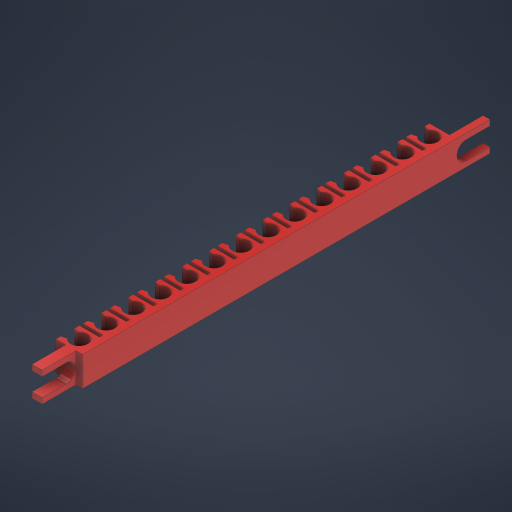
# Autodesk Inventor part: Hose Clamp
Saved by Autodesk Inventor 2024 (Build 280153000, 153)
## iProperties
Created: 2023-05-24
Part Number: Hose Clamp
Material: Generic
Document SubType Name: Modeling
Designer: cfangmeier3
Density: 1 g/cm^3
Appearance: Default
Author: cfangmeier3
Autodesk Inventor part; units mm, degrees
ref_plane "YZ Plane" through (0, 0, 0) normal (1, 0, 0) x (0, 1, 0)
ref_plane "XZ Plane" through (0, 0, 0) normal (0, 1, 0) x (-1, 0, 0)
ref_plane "XY Plane" through (0, 0, 0) normal (0, 0, 1) x (1, 0, 0)
sketch "Sketch1" plane through (0, 0, 0) normal (0, 1, 0) x (-1, 0, 0)
  line L0 (0, 71.12) -> (0, -71.12)
  line L1 (2.54, 71.12) -> (10.0965, 71.12)
  line L2 (10.0965, 71.12) -> (10.0965, 69.215)
  line L3 (10.0965, 64.135) -> (10.0965, 62.23)
  line L4 (10.0965, 69.215) -> (8.1249, 68.7234)
  line L5 (10.0965, 64.135) -> (8.1249, 64.6266)
  arc A0 (8.1249, 68.7234) -> (8.1249, 64.6266) centre (5.699, 66.675) ccw
  line L6 (10.0965, 62.23) -> (2.54, 62.23)
  line L7 (2.54, 62.23) -> (2.54, 60.96)
  line L8 (2.54, 52.07) -> (2.54, 50.8)
  line L9 (10.0965, 52.07) -> (2.54, 52.07)
  line L10 (10.0965, 53.975) -> (10.0965, 52.07)
  line L11 (10.0965, 59.055) -> (8.1249, 58.5634)
  arc A1 (8.1249, 58.5634) -> (8.1249, 54.4666) centre (5.699, 56.515) ccw
  line L12 (2.54, 60.96) -> (10.0965, 60.96)
  line L13 (10.0965, 60.96) -> (10.0965, 59.055)
  line L14 (10.0965, 53.975) -> (8.1249, 54.4666)
  line L15 (2.54, 41.91) -> (2.54, 40.64)
  line L16 (10.0965, 41.91) -> (2.54, 41.91)
  line L17 (10.0965, 43.815) -> (10.0965, 41.91)
  line L18 (10.0965, 48.895) -> (8.1249, 48.4034)
  arc A2 (8.1249, 48.4034) -> (8.1249, 44.3066) centre (5.699, 46.355) ccw
  line L19 (2.54, 50.8) -> (10.0965, 50.8)
  line L20 (10.0965, 50.8) -> (10.0965, 48.895)
  line L21 (10.0965, 43.815) -> (8.1249, 44.3066)
  line L22 (2.54, 31.75) -> (2.54, 30.48)
  line L23 (10.0965, 31.75) -> (2.54, 31.75)
  line L24 (10.0965, 33.655) -> (10.0965, 31.75)
  line L25 (10.0965, 38.735) -> (8.1249, 38.2434)
  arc A3 (8.1249, 38.2434) -> (8.1249, 34.1466) centre (5.699, 36.195) ccw
  line L26 (2.54, 40.64) -> (10.0965, 40.64)
  line L27 (10.0965, 40.64) -> (10.0965, 38.735)
  line L28 (10.0965, 33.655) -> (8.1249, 34.1466)
  line L29 (2.54, 21.59) -> (2.54, 20.32)
  line L30 (10.0965, 21.59) -> (2.54, 21.59)
  line L31 (10.0965, 23.495) -> (10.0965, 21.59)
  line L32 (10.0965, 28.575) -> (8.1249, 28.0834)
  arc A4 (8.1249, 28.0834) -> (8.1249, 23.9866) centre (5.699, 26.035) ccw
  line L33 (2.54, 30.48) -> (10.0965, 30.48)
  line L34 (10.0965, 30.48) -> (10.0965, 28.575)
  line L35 (10.0965, 23.495) -> (8.1249, 23.9866)
  line L36 (2.54, 11.43) -> (2.54, 10.16)
  line L37 (10.0965, 11.43) -> (2.54, 11.43)
  line L38 (10.0965, 13.335) -> (10.0965, 11.43)
  line L39 (10.0965, 18.415) -> (8.1249, 17.9234)
  arc A5 (8.1249, 17.9234) -> (8.1249, 13.8266) centre (5.699, 15.875) ccw
  line L40 (2.54, 20.32) -> (10.0965, 20.32)
  line L41 (10.0965, 20.32) -> (10.0965, 18.415)
  line L42 (10.0965, 13.335) -> (8.1249, 13.8266)
  line L43 (2.54, 1.27) -> (2.54, 0)
  line L44 (10.0965, 1.27) -> (2.54, 1.27)
  line L45 (10.0965, 3.175) -> (10.0965, 1.27)
  line L46 (10.0965, 8.255) -> (8.1249, 7.7634)
  arc A6 (8.1249, 7.7634) -> (8.1249, 3.6666) centre (5.699, 5.715) ccw
  line L47 (2.54, 10.16) -> (10.0965, 10.16)
  line L48 (10.0965, 10.16) -> (10.0965, 8.255)
  line L49 (10.0965, 3.175) -> (8.1249, 3.6666)
  line L50 (2.54, -8.89) -> (2.54, -10.16)
  line L51 (10.0965, -8.89) -> (2.54, -8.89)
  line L52 (10.0965, -6.985) -> (10.0965, -8.89)
  line L53 (10.0965, -1.905) -> (8.1249, -2.3966)
  arc A7 (8.1249, -2.3966) -> (8.1249, -6.4934) centre (5.699, -4.445) ccw
  line L54 (2.54, 0) -> (10.0965, 0)
  line L55 (10.0965, 0) -> (10.0965, -1.905)
  line L56 (10.0965, -6.985) -> (8.1249, -6.4934)
  line L57 (2.54, -19.05) -> (2.54, -20.32)
  line L58 (10.0965, -19.05) -> (2.54, -19.05)
  line L59 (10.0965, -17.145) -> (10.0965, -19.05)
  line L60 (10.0965, -12.065) -> (8.1249, -12.5566)
  arc A8 (8.1249, -12.5566) -> (8.1249, -16.6534) centre (5.699, -14.605) ccw
  line L61 (2.54, -10.16) -> (10.0965, -10.16)
  line L62 (10.0965, -10.16) -> (10.0965, -12.065)
  line L63 (10.0965, -17.145) -> (8.1249, -16.6534)
  line L64 (2.54, -29.21) -> (2.54, -30.48)
  line L65 (10.0965, -29.21) -> (2.54, -29.21)
  line L66 (10.0965, -27.305) -> (10.0965, -29.21)
  line L67 (10.0965, -22.225) -> (8.1249, -22.7166)
  arc A9 (8.1249, -22.7166) -> (8.1249, -26.8134) centre (5.699, -24.765) ccw
  line L68 (2.54, -20.32) -> (10.0965, -20.32)
  line L69 (10.0965, -20.32) -> (10.0965, -22.225)
  line L70 (10.0965, -27.305) -> (8.1249, -26.8134)
  line L71 (2.54, -39.37) -> (2.54, -40.64)
  line L72 (10.0965, -39.37) -> (2.54, -39.37)
  line L73 (10.0965, -37.465) -> (10.0965, -39.37)
  line L74 (10.0965, -32.385) -> (8.1249, -32.8766)
  arc A10 (8.1249, -32.8766) -> (8.1249, -36.9734) centre (5.699, -34.925) ccw
  line L75 (2.54, -30.48) -> (10.0965, -30.48)
  line L76 (10.0965, -30.48) -> (10.0965, -32.385)
  line L77 (10.0965, -37.465) -> (8.1249, -36.9734)
  line L78 (2.54, -49.53) -> (2.54, -50.8)
  line L79 (10.0965, -49.53) -> (2.54, -49.53)
  line L80 (10.0965, -47.625) -> (10.0965, -49.53)
  line L81 (10.0965, -42.545) -> (8.1249, -43.0366)
  arc A11 (8.1249, -43.0366) -> (8.1249, -47.1334) centre (5.699, -45.085) ccw
  line L82 (2.54, -40.64) -> (10.0965, -40.64)
  line L83 (10.0965, -40.64) -> (10.0965, -42.545)
  line L84 (10.0965, -47.625) -> (8.1249, -47.1334)
  line L85 (2.54, -59.69) -> (2.54, -60.96)
  line L86 (10.0965, -59.69) -> (2.54, -59.69)
  line L87 (10.0965, -57.785) -> (10.0965, -59.69)
  line L88 (10.0965, -52.705) -> (8.1249, -53.1966)
  arc A12 (8.1249, -53.1966) -> (8.1249, -57.2934) centre (5.699, -55.245) ccw
  line L89 (2.54, -50.8) -> (10.0965, -50.8)
  line L90 (10.0965, -50.8) -> (10.0965, -52.705)
  line L91 (10.0965, -57.785) -> (8.1249, -57.2934)
  line L92 (2.54, -69.85) -> (2.54, -71.12)
  line L93 (10.0965, -69.85) -> (2.54, -69.85)
  line L94 (10.0965, -67.945) -> (10.0965, -69.85)
  line L95 (10.0965, -62.865) -> (8.1249, -63.3566)
  arc A13 (8.1249, -63.3566) -> (8.1249, -67.4534) centre (5.699, -65.405) ccw
  line L96 (2.54, -60.96) -> (10.0965, -60.96)
  line L97 (10.0965, -60.96) -> (10.0965, -62.865)
  line L98 (10.0965, -67.945) -> (8.1249, -67.4534)
  line L99 (0, 71.12) -> (2.54, 71.12)
  line L100 (6.35, 71.12) -> (2.54, 71.12)
  line L101 (2.54, 71.12) -> (2.54, 83.82)
  line L102 (2.54, 83.82) -> (6.35, 83.82)
  line L103 (6.35, 83.82) -> (6.35, 71.12)
  line L104 (2.54, -71.12) -> (2.54, -82.55)
  line L105 (2.54, -82.55) -> (0, -82.55)
  line L106 (0, -82.55) -> (0, -71.12)
  point P0 (0, 0)
  dimension "d1" = 7.5565
  dimension "d5" = 104
  dimension "d6" = 104
  dimension "d7" = 3.175
  dimension "d8" = 2.032
  dimension "d9" = 2.54
  dimension "d10" = 1.27
  dimension "d11" = 8.89
  dimension "d12" = 1.905
  dimension "d16" = 10.16
  dimension "d25" = 142.24
  dimension "d26" = 71.12
  dimension "d27" = 12.7
  dimension "d28" = 3.81
  dimension "d29" = 2.54
  dimension "d41" = 12.7
  constraints: 214 end point, 28 point on circle, 14 centre point, 6 vertical, 4 horizontal, 3 perpendicular, 2 equal length, 2 horizontal alignment, 2 parallel, 1 midpoint, 1 point on line, 1 vertical alignment, 234 other
  measures "d1" distance of L1.start L1.end
  measures "d5" angle of L4 L2
  measures "d6" angle of L5 L3
  measures "d7" radius of A0
  measures "d8" distance of L2.end L4.end
  measures "d9" distance from line of L0 L6.end
  measures "d10" distance of L6.end L7.end
  measures "d11" distance between parallel lines of L1 L6
  measures "d12" distance of L1.end L2.end
  measures "d16" distance of L7.end L8.end
  measures "d25" distance of L0.start L0.end
  measures "d26" distance of L0.end point (0, 0)
  measures "d27" distance of L102.end L100.start
  measures "d28" distance of L101.end L102.end
  measures "d29" distance of L0.start L100.end
  measures "d41" distance between parallel lines of L105 L93
extrude "Extrusion1" add sketch "Sketch1" along normal blind 11.1125
sketch "Sketch3" plane through (0, 0, 71.12) normal (1, 0, 0) x (0, 0, -1)
  line L0 (162.687, 5.5563) -> (144.653, 5.5562) construction
  line L1 (162.687, 8.9853) -> (144.653, 8.9853)
  line L2 (144.653, 2.1272) -> (162.687, 2.1273)
  arc A0 (162.687, 2.1273) -> (162.687, 8.9853) centre (162.687, 5.5563) ccw
  arc A1 (144.653, 8.9853) -> (144.653, 2.1272) centre (144.653, 5.5562) ccw
  line L3 (153.67, 0) -> (153.67, 11.1125) projected
  line L4 (0, 11.1125) -> (153.67, 11.1125) projected
  line L5 (-21.717, 5.5563) -> (-3.683, 5.5563) construction
  line L6 (-21.717, 2.1273) -> (-3.683, 2.1273)
  line L7 (-3.683, 8.9853) -> (-21.717, 8.9852)
  arc A2 (-21.717, 8.9852) -> (-21.717, 2.1273) centre (-21.717, 5.5563) ccw
  arc A3 (-3.683, 2.1273) -> (-3.683, 8.9853) centre (-3.683, 5.5563) ccw
  line L8 (-12.7, 0) -> (-12.7, 11.1125) projected
  point P0 (71.12, 0)
  point P1 (153.67, 5.5563)
  point P2 (-12.7, 5.5563)
  point P3 (-12.7, 8.9853)
  point P4 (-12.7, 2.1273)
  point P5 (153.67, 2.1273)
  point P6 (153.67, 8.9853)
  dimension "d45" = 11.1125
  dimension "d46" = 5.5563
  dimension "d47" = 9.017
  dimension "d48" = 9.017
  dimension "d49" = 6.858
  dimension "d50" = 6.858
  constraints: 16 end point, 8 point on circle, 8 tangent, 4 centre point, 3 midpoint, 2 horizontal, 2 parallel, 1 collinear, 1 horizontal alignment
  measures "d45" distance of L3.start L3.end
  measures "d46" distance from line of L4 point (153.67, 5.556)
  measures "d47" distance from line of L3 L0.end
  measures "d48" distance from line of L8 L5.end
  measures "d49" distance between parallel lines of L1 L2
  measures "d50" distance between parallel lines of L7 L6
extrude "Extrusion2" cut sketch "Sketch3" against normal through all contours L3 L2 A1 L1 | L8 L7 A3 L6
equation "\"d6\" = d5"
body "Solid1"
